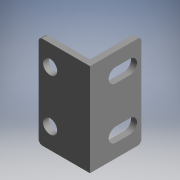
# Autodesk Inventor part: HPTBD5-SEP_b.
Saved by Autodesk Inventor 2017.3 (Build 213256000, 256)
## iProperties
Part Number: HPTBD5-SEP_b.
Material: Generic
Catalog Web Link: www.cadenas.de
Description: HPTBS5, SHPTBS5, HPTBD5, SHPTBD5, HPTBDW5, SHPTBDW5, HPTGS5_body-Sheet Metal Brackets - For HFS5 Series - Bent Type
Vendor: MISUMI
Document SubType Name: Modeling
Designer: partserver
Manufacturer: MISUMI
Mass: 2.75939 g
Surface Area: 29.4213 cm^2
Volume: 2.75939 cm^3
Density: 1 g/cm^3
Appearance: PSOLRGB-175-175-175
Category: PARTsolutions
Company: MISUMI
Title: HPTBD5-SEP
Author: Cadenas PARTsolutions
Comments: Sheet Metal Brackets - For HFS5 Series - Bent Type
PSOL_IDENT_0: {$CADENAS_DATA\23d-libs\misumi\metric\38_al_extrusions_blackets\5\hptbs5\hptbs5.prj},239 {VTYP=3D},{
PSOL_IDENT_1: NB=HPTBD5-SEP_b.},{LINA=HPTBD5-SEP},{NN=HPTBS5, SHPTBS5, HPTBD5, SHPTBD5, HPTBDW5, SHPTBDW5, HPTGS5_
PSOL_IDENT_2: body},{DATE=08.06.2021 08:25:19},{GEOMDATE=24.03.2020 04:31:18},{VERSION=},{LINEID=270},{WBVAR=MAT,S
PSOL_IDENT_3: HPT,NOH,ALT1},{WBNUMERIC=}  {NB=HPTBD5-SEP_b.},{LINA=HPTBD5-SEP},{KT=5},{PN=HPTBD5-SEP},{TYPE=HPTBD}
PSOL_IDENT_4: ,{NO=5},{MAT=},{ST=Bright Chromate},{SHPT=L},{SHPTALG= 'L', 'L-Shaped Bent','B', 'Both Ends Bemt' },
PSOL_IDENT_5: {NOH=BD},{NOHALG= 'BS','2','BD','4','BDW','8' },{MASS=21},{A=36},{B=20},{T=2.3},{N=5.5},{E=15.5},{W=
PSOL_IDENT_6: 20},{H=10.0},{G=5.5},{F=0},{R=1.5},{ALT1=-SEP},{AB=CBM5-8},{ABD=5},{ABL=8},{NOB=4},{AN=HNTP5-5},{NON=
PSOL_IDENT_7: 4},{AB1=5-8},{AN1=5-5},{MAT1='', 'Low Carbon Steel', 'S', '304 Stainless Steel'},{NUTMAT=1010 Carbon
PSOL_IDENT_8: Steel Equivalent},{NUTTHREAD=5},{NUT1=5},{C=3.000}
NB: HPTBD5-SEP_b.
NN: HPTBS5, SHPTBS5, HPTBD5, SHPTBD5, HPTBDW5, SHPTBDW5, HPTGS5_body
NT: Sheet Metal Brackets - For HFS5 Series - Bent Type
NBSYN: $PN._b.
LINA: HPTBD5-SEP
CATALOG: Misumi
PN: HPTBD5-SEP
NO: 5
MAT: Low Carbon Steel
ST: Bright Chromate
SHPT: L-Shaped Bent
NOH: 4
MASS: 21
T: 2.3
ALT1: with SEP (Post-Assembly Fitting Spring Nuts Set of Applicable Bolt and Nut)
AB: CBM5-8
NOB: 4
AN: HNTP5-5
NON: 4
SUPPLIER: MISUMI
ARTICLENO: HPTBD5-SEP_b.
BOMINFO: HPTBD5-SEP
CREATOR: CADENAS GmbH
Autodesk Inventor part; units mm, degrees
sketch "Sketch_2" plane through (0, 0, 0) normal (0, 1, 0) x (-1, 0, 0)
  line L0 (0, 18) -> (-18.5, 18)
  arc A0 (-18.5, 18) -> (-20, 16.5) centre (-18.5, 16.5) ccw
  line L1 (-20, 16.5) -> (-20, -16.5)
  arc A1 (-20, -16.5) -> (-18.5, -18) centre (-18.5, -16.5) ccw
  line L2 (-18.5, -18) -> (0, -18)
  line L3 (0, -18) -> (0, 18)
  circle A2 centre (-15.5, -10) radius 2.75
  circle A3 centre (-15.5, 10) radius 2.75
  constraints: 8 end point, 4 centre point, 4 point on circle
extrude "Extrusion1" add sketch "Sketch_2" along normal blind 2.3
sketch "Sketch_1" plane through (0, 0, 0) normal (1, 0, 0) x (0, 1, 0)
  line L0 (18.5, 18) -> (0, 18)
  line L1 (0, 18) -> (0, -18)
  line L2 (0, -18) -> (18.5, -18)
  arc A0 (18.5, -18) -> (20, -16.5) centre (18.5, -16.5) ccw
  line L3 (20, -16.5) -> (20, 16.5)
  arc A1 (20, 16.5) -> (18.5, 18) centre (18.5, 16.5) ccw
  line L4 (15.5, -7.25) -> (10, -7.25)
  arc A2 (10, -7.25) -> (10, -12.75) centre (10, -10) ccw
  line L5 (10, -12.75) -> (15.5, -12.75)
  arc A3 (15.5, -12.75) -> (15.5, -7.25) centre (15.5, -10) ccw
  line L6 (15.5, 12.75) -> (10, 12.75)
  arc A4 (10, 12.75) -> (10, 7.25) centre (10, 10) ccw
  line L7 (10, 7.25) -> (15.5, 7.25)
  arc A5 (15.5, 7.25) -> (15.5, 12.75) centre (15.5, 10) ccw
  constraints: 16 end point, 12 point on circle, 6 centre point
extrude "Extrusion2" add sketch "Sketch_1" along normal blind 2.3
ref_plane "to_cbm_1_1_XY" through (2.3, 15.5, -10) normal (1, 0, 0) x (0, 0, -1)
ref_plane "to_cbm_1_1_YZ" through (2.3, 15.5, -10) normal (0, 0, -1) x (0, 1, 0)
ref_plane "to_cbm_1_1_ZX" through (2.3, 15.5, -10) normal (0, 1, 0) x (1, 0, 0)
ref_plane "to_cbm_1_2_XY" through (2.3, 15.5, 10) normal (1, 0, 0) x (0, 0, -1)
ref_plane "to_cbm_1_2_YZ" through (2.3, 15.5, 10) normal (0, 0, -1) x (0, 1, 0)
ref_plane "to_cbm_1_2_ZX" through (2.3, 15.5, 10) normal (0, 1, 0) x (1, 0, 0)
ref_plane "to_cbm_2_1_XY" through (15.5, 2.3, 10) normal (0, 1, 0) x (1, 0, 0)
ref_plane "to_cbm_2_1_YZ" through (15.5, 2.3, 10) normal (1, 0, 0) x (0, 0, -1)
ref_plane "to_cbm_2_1_ZX" through (15.5, 2.3, 10) normal (0, 0, -1) x (0, 1, 0)
ref_plane "to_cbm_2_2_XY" through (15.5, 2.3, -10) normal (0, 1, 0) x (1, 0, 0)
ref_plane "to_cbm_2_2_YZ" through (15.5, 2.3, -10) normal (1, 0, 0) x (0, 0, -1)
ref_plane "to_cbm_2_2_ZX" through (15.5, 2.3, -10) normal (0, 0, -1) x (0, 1, 0)
ref_plane "to_hntp5_1_1_XY" through (-2, 15.5, -10) normal (-1, 0, 0) x (0, -1, 0)
ref_plane "to_hntp5_1_1_YZ" through (-2, 15.5, -10) normal (0, -1, 0) x (0, 0, 1)
ref_plane "to_hntp5_1_1_ZX" through (-2, 15.5, -10) normal (0, 0, 1) x (-1, 0, 0)
ref_plane "to_hntp5_1_2_XY" through (-2, 15.5, 10) normal (-1, 0, 0) x (0, -1, 0)
ref_plane "to_hntp5_1_2_YZ" through (-2, 15.5, 10) normal (0, -1, 0) x (0, 0, 1)
ref_plane "to_hntp5_1_2_ZX" through (-2, 15.5, 10) normal (0, 0, 1) x (-1, 0, 0)
ref_plane "to_hntp5_2_1_XY" through (15.5, -2, 10) normal (0, -1, 0) x (-1, 0, 0)
ref_plane "to_hntp5_2_1_YZ" through (15.5, -2, 10) normal (-1, 0, 0) x (0, 0, -1)
ref_plane "to_hntp5_2_1_ZX" through (15.5, -2, 10) normal (0, 0, -1) x (0, -1, 0)
ref_plane "to_hntp5_2_2_XY" through (15.5, -2, -10) normal (0, -1, 0) x (-1, 0, 0)
ref_plane "to_hntp5_2_2_YZ" through (15.5, -2, -10) normal (-1, 0, 0) x (0, 0, -1)
ref_plane "to_hntp5_2_2_ZX" through (15.5, -2, -10) normal (0, 0, -1) x (0, -1, 0)
body "Solid1"
